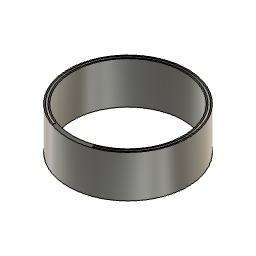
Mid Joint v4 (Autodesk Fusion 360 design; units mm, degrees)
Autodesk Fusion 360 part; units mm, degrees
sketch "Sketch1" plane through (0, 0, 0) normal (0, 0, 1) x (1, 0, 0)
  circle A0 centre (0, 0) radius 60
  circle A1 centre (0, 0) radius 58
  circle A2 centre (0, 0) radius 60.5
  circle A3 centre (0, 0) radius 62.5
  dimension "d1" = 120
  dimension "d2" = 116
  dimension "d3" = 121
  dimension "d4" = 125
  constraint coincident A0.centre A1.centre
  constraint concentric A0 A1
  measures "d1" diameter of A0
  measures "d2" diameter of A1
  measures "d3" diameter of A2
  measures "d4" diameter of A3
extrude "Extrude1" add sketch "Sketch1" along normal blind 20 makes body 1 at (59.9254, -2.9908, 13.3333) makes body 2 at (62.4223, -3.1154, 13.3333)
sketch "Sketch2" plane through (0, 0, 0) normal (0, 0, -1) x (1, 0, 0)
  circle A0 centre (0, 0) radius 58
  circle A1 centre (0, 0) radius 60
  circle A2 centre (0, 0) radius 60
  circle A3 centre (0, 0) radius 60.5
  dimension "d11" = 120
  dimension "d12" = 121
  constraint coincident A0.centre A1.centre
  measures "d11" diameter of A2
  measures "d12" diameter of A3
extrude "Extrude2" add sketch "Sketch1" against normal blind 4 contours A0 | A2 | A3 bodies 2 1
sketch "Sketch3" plane through (0, 0, -4) normal (0, 0, -1) x (1, 0, 0)
  circle A0 centre (0, 0) radius 58
  circle A1 centre (0, 0) radius 62.5
  circle A2 centre (0, 0) radius 58
  circle A3 centre (0, 0) radius 60
  circle A4 centre (0, 0) radius 60.5
  circle A5 centre (0, 0) radius 62.5
  dimension "d13" = 116
  dimension "d14" = 120
  dimension "d15" = 121
  dimension "d16" = 125
  constraint coincident A0.centre A1.centre
  constraint concentric A3 A4
  constraint concentric A3 A5
  measures "d13" diameter of A2
  measures "d14" diameter of A3
  measures "d15" diameter of A4
  measures "d16" diameter of A5
extrude "Extrude4" add sketch "Sketch3" along normal blind 20 bodies 2
sketch "Sketch4" plane through (0, 0, 20) normal (0, 0, 1) x (-1, 0, 0)
  circle A0 centre (0, 0) radius 60.5
  circle A1 centre (0, 0) radius 62.5
  line L0 (0, 0) -> (0, 62.5)
  line L1 (0, 0) -> (-20.5, 0)
  line L2 (0, 62.5) -> (20.5, 62.5)
  line L3 (-20.5, 0) -> (20.5, 0)
  line L4 (20.5, 0) -> (20.5, 62.5)
  line L5 (20.5, 62.5) -> (-20.5, 62.5)
  line L6 (-20.5, 62.5) -> (-20.5, 0)
  circle A2 centre (0, 0) radius 60
  dimension "d19" = 20.5
  dimension "d21" = 20.5
  dimension "d22" = 120
  constraint coincident A0.centre A1.centre
  constraint coincident A1 L0.end
  constraint vertical L0
  constraint perpendicular L0 L1
  constraint perpendicular L0 L2
  constraint horizontal L3
  constraint vertical L4
  constraint horizontal L5
  constraint vertical L6
  measures "d19" distance of A0.centre L1.end
  measures "d21" distance of L0.end L2.end
  measures "d22" diameter of A2
extrude "Extrude5" add sketch "Sketch4" against normal blind 20 contours A0 L0 L4 A2 | A0 L0 L6 A2 bodies 2
copy_body "Body->Comp1" bodies 2 removing the originals makes body 3 in component "midjoint"
sketch "Sketch5" plane through (0, 0, -24) normal (0, 0, -1) x (1, 0, 0)
  circle A0 centre (0, 0) radius 58
  circle A1 centre (0, 0) radius 60
  circle A2 centre (0, 0) radius 59.25
  circle A3 centre (0, 0) radius 61.25
  dimension "d35" = 118.5
  dimension "d36" = 122.5
  constraint coincident A0.centre A1.centre
  measures "d35" diameter of A2
  measures "d36" diameter of A3
extrude "Extrude1'" cut sketch "Sketch5" against normal blind 20 contours A1 | A3 bodies 3 in component "midjoint"
sketch "Sketch6" plane through (0, 0, 20) normal (0, 0, 1) x (-1, 0, 0)
  circle A0 centre (0, 0) radius 62.5
  circle A1 centre (0, 0) radius 58
  arc A2 (-20.5, 56.3893) -> (20.5, 56.3893) centre (0, 0) ccw
  line L0 (20.5, 56.3893) -> (20.5, 56.921)
  arc A3 (-20.5, 56.921) -> (20.5, 56.921) centre (0, 0) ccw
  line L1 (-20.5, 56.921) -> (-20.5, 56.3893)
  circle A4 centre (0, 0) radius 59.25
  circle A5 centre (-0.0055, -0.0156) radius 61.25
  line L2 (20.5, 56.921) -> (20.5, 57.7)
  line L3 (20.5, 56.3893) -> (20.5, 55.5906)
  line L4 (-20.5, 56.921) -> (-20.5, 57.7039)
  line L5 (-20.5, 56.3893) -> (-20.5, 55.5906)
  dimension "d33" = 118.5
  dimension "d34" = 122.5
  constraint concentric A0 A4
  constraint coincident L0.end A3.end
  constraint coincident A5 L2.end
  constraint parallel L0 L2
  constraint coincident A2.end L0.start
  constraint coincident A4 L3.end
  constraint parallel L0 L3
  constraint coincident A3.start L1.start
  constraint coincident A5 L4.end
  constraint parallel L1 L4
  constraint coincident A2.start L1.end
  constraint coincident A4 L5.end
  constraint parallel L1 L5
  measures "d33" diameter of A4
  measures "d34" diameter of A5
extrude "Extrude2'" cut sketch "Sketch6" against normal blind 20 contours A2 A4 L3 L5 | A2 L0 A3 L1 | A3 A5 L2 L4 bodies 3 in component "midjoint"
component "midjoint" placed x (1, 0, 0) y (0, 1, 0) z (0, 0, 1) at (0, 0, 0)
named bodies: "midjoint"
